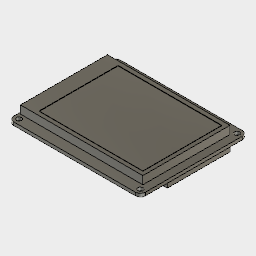
3315 2.4in TFT Feather Wing (Autodesk Fusion 360 design; units mm, degrees)
Autodesk Fusion 360 part; units mm, degrees
note: some values were not read from the file. Set by a fixed rule: which sketch regions a step uses.
sketch "pcb" plane through (0, 0, 0) normal (0, 0, 1) x (1, 0, 0)
  line L0 (0, 0) -> (64.77, 0)
  line L1 (64.77, 0) -> (64.77, 52.578)
  line L2 (64.77, 52.578) -> (0, 52.578)
  line L3 (0, 52.578) -> (0, 0)
  circle A0 centre (2.54, 50.038) radius 1.27
  line L4 (32.385, 52.578) -> (32.385, 0) construction
  line L5 (0, 26.289) -> (64.77, 26.289) construction
  circle A1 centre (62.23, 50.038) radius 1.27
  circle A2 centre (2.54, 2.54) radius 1.27
  circle A3 centre (62.23, 2.54) radius 1.27
  dimension "d1" = 64.77
  dimension "d2" = 52.578
  dimension "d3" = 2.54
  dimension "d4" = 2.54
  dimension "d5" = 2.54
  measures "d1" distance of L1.end L2.end
  measures "d2" distance of L0.start L2.end
  measures "d3" diameter of A0
  measures "d4" distance of L3 A0.centre
  measures "d5" distance of L2 A0.centre
extrude "Extrude1" add sketch "pcb" along normal blind 1.6 makes body 1
fillet "Fillet1" radius 2.54 4 edges at (64.77, 0, 0.8) (0, 0, 0.8) (0, 52.578, 0.8) (64.77, 52.578, 0.8) on bodies 1
sketch "bottom" plane through (0, 0, 0) normal (0, 0, -1) x (1, 0, 0)
  circle A0 centre (62.23, -50.038) radius 1.27
  circle A1 centre (2.54, -2.54) radius 1.27
  circle A2 centre (62.23, -2.54) radius 1.27
  circle A3 centre (2.54, -50.038) radius 1.27
  arc A4 (62.23, -52.578) -> (64.77, -50.038) centre (62.23, -50.038) ccw
  line L0 (64.77, -50.038) -> (64.77, -2.54)
  arc A5 (64.77, -2.54) -> (62.23, 0) centre (62.23, -2.54) ccw
  line L1 (62.23, 0) -> (2.54, 0)
  arc A6 (2.54, 0) -> (0, -2.54) centre (2.54, -2.54) ccw
  line L2 (0, -2.54) -> (0, -50.038)
  arc A7 (0, -50.038) -> (2.54, -52.578) centre (2.54, -50.038) ccw
  line L3 (2.54, -52.578) -> (62.23, -52.578)
  line L4 (62.97, -45.978) -> (57.97, -45.978)
  line L5 (57.97, -45.978) -> (57.97, -14.978)
  line L6 (57.97, -14.978) -> (62.97, -14.978)
  line L7 (62.97, -14.978) -> (62.97, -45.978)
  line L8 (40.17, -45.978) -> (35.17, -45.978)
  line L9 (35.17, -45.978) -> (35.17, -4.978)
  line L10 (35.17, -4.978) -> (40.17, -4.978)
  line L11 (40.17, -4.978) -> (40.17, -45.978)
  line L12 (1.6, -6.8) -> (7.6, -6.8)
  line L13 (7.6, -6.8) -> (7.6, -12.8)
  line L14 (7.6, -12.8) -> (1.6, -12.8)
  line L15 (1.6, -12.8) -> (1.6, -6.8)
  line L16 (1.6, -6.8) -> (7.6, -12.8) construction
  line L17 (7.6, -6.8) -> (1.6, -12.8) construction
  circle A8 centre (4.6, -9.8) radius 1.5
  line L18 (5.5, -17.4) -> (2, -17.4)
  line L19 (2, -17.4) -> (2, -24.4)
  line L20 (2, -24.4) -> (5.5, -24.4)
  line L21 (5.5, -24.4) -> (5.5, -17.4)
  line L22 (15.5, -43.978) -> (0, -43.978)
  line L23 (0, -43.978) -> (0, -29.978)
  line L24 (0, -29.978) -> (15.5, -29.978)
  line L25 (15.5, -29.978) -> (15.5, -43.978)
  point P0 (4.6, -9.8)
  dimension "d9" = 5
  dimension "d10" = 5
  dimension "d11" = 31
  dimension "d12" = 41
  dimension "d13" = 6.6
  dimension "d14" = 6.6
  dimension "d15" = 1.8
  dimension "d16" = 17.8
  dimension "d19" = 6
  dimension "d20" = 6
  dimension "d21" = 6.8
  dimension "d22" = 1.6
  dimension "d23" = 3
  dimension "d28" = 3.5
  dimension "d29" = 7
  dimension "d30" = 2
  dimension "d31" = 17.4
  dimension "d32" = 15.5
  dimension "d33" = 14
  dimension "d34" = 8.6
  measures "d9" distance of L5.end L6.end
  measures "d10" distance of L9.end L10.end
  measures "d11" distance of L4.start L6.end
  measures "d12" distance of L8.start L10.end
  measures "d13" distance of L3 L4
  measures "d14" distance of L3 L8
  measures "d15" distance of L0 L7
  measures "d16" distance of L5 L11
  measures "d19" distance of L13.end L14.end
  measures "d20" distance of L12.end L13.end
  measures "d21" distance of L1 L12
  measures "d22" distance of L2 L15
  measures "d23" diameter of A8
  measures "d28" distance of L18.start L18.end
  measures "d29" distance of L18.start L20.end
  measures "d30" distance of L2 L19
  measures "d31" distance of L1 L18
  measures "d32" distance of L22.start L22.end
  measures "d33" distance of L22.start L24.end
  measures "d34" distance of L3 L22
extrude "Extrude2" add sketch "bottom" along normal blind 3.9 separate body contours L4 L5 L6 L7 | L8 L9 L10 L11 makes body 2 at (61.3033, 25.3113, 0) makes body 3 at (38.5033, 32.3113, 0)
extrude "Extrude3" add sketch "bottom" along normal blind 1.8 separate body contours L12 L13 L14 L15 | A8 makes body 4
extrude "Extrude4" add sketch "bottom" along normal blind 3 contours A8 bodies 4
extrude "Extrude5" add sketch "bottom" along normal blind 1.4 separate body contours L18 L19 L20 L21 makes body 5
extrude "Extrude6" add sketch "bottom" along normal blind 1.7 separate body contours L2 L22 L23 L24 L25 makes body 6
sketch "microSD" plane through (0, 0, -1.7) normal (0, 0, -1) x (1, 0, 0)
  line L0 (15.5, -29.978) -> (0, -29.978)
  line L1 (0, -29.978) -> (0, -43.978)
  line L2 (0, -43.978) -> (15.5, -43.978)
  line L3 (15.5, -43.978) -> (15.5, -29.978)
  circle A0 centre (-8.5, -35.5) radius 11
  dimension "d39" = 22
  measures "d39" diameter of A0
extrude "Extrude7" cut sketch "microSD" against normal blind 1.7 contours L0 L1 A0 picked at (0.2923, -37.9037) bodies 6
sketch "switch" plane through (0, 0, -1.4) normal (0, 0, -1) x (1, 0, 0)
  line L0 (5.5, -24.4) -> (5.5, -17.4)
  line L1 (5.5, -17.4) -> (2, -17.4)
  line L2 (2, -17.4) -> (2, -24.4)
  line L3 (2, -24.4) -> (5.5, -24.4)
  line L4 (2, -20.9) -> (5.5, -20.9)
  line L5 (2, -19.4) -> (3, -19.4)
  line L6 (3, -19.4) -> (3, -22.4)
  line L7 (3, -22.4) -> (2, -22.4)
  line L8 (2, -22.4) -> (2, -19.4)
  line L9 (3, -20.9) -> (2, -20.9) construction
  dimension "d42" = 3
  dimension "d43" = 1
  measures "d42" distance of L5.end L6.end
  measures "d43" distance of L6.end L7.end
extrude "Extrude8" add sketch "switch" along normal blind 1 contours L2 L4 L6 L7 L8 bodies 5
sketch "display" plane through (0, 0, 1.6) normal (0, 0, 1) x (-1, 0, 0)
  arc A0 (-64.77, -50.038) -> (-62.23, -52.578) centre (-62.23, -50.038) ccw
  line L0 (-62.23, -52.578) -> (-2.54, -52.578)
  arc A1 (-2.54, -52.578) -> (0, -50.038) centre (-2.54, -50.038) ccw
  line L1 (0, -50.038) -> (0, -2.54)
  arc A2 (0, -2.54) -> (-2.54, 0) centre (-2.54, -2.54) ccw
  line L2 (-2.54, 0) -> (-62.23, 0)
  arc A3 (-62.23, 0) -> (-64.77, -2.54) centre (-62.23, -2.54) ccw
  line L3 (-64.77, -2.54) -> (-64.77, -50.038)
  circle A4 centre (-62.23, -50.038) radius 1.27
  circle A5 centre (-2.54, -2.54) radius 1.27
  circle A6 centre (-62.23, -2.54) radius 1.27
  circle A7 centre (-2.54, -50.038) radius 1.27
  line L4 (-0.8, -47.778) -> (-61, -47.778)
  line L5 (-61, -47.778) -> (-61, -4.978)
  line L6 (-61, -4.978) -> (-0.8, -4.978)
  line L7 (-0.8, -4.978) -> (-0.8, -47.778)
  dimension "d46" = 60.2
  dimension "d47" = 42.8
  dimension "d48" = 4.8
  dimension "d49" = 0.8
  measures "d46" distance of L4.start L4.end
  measures "d47" distance of L4.start L6.end
  measures "d48" distance of L0 L4
  measures "d49" distance of L1 L7
extrude "Extrude9" add sketch "display" along normal blind 3.9 separate body contours L4 L5 L6 L7 makes body 7
sketch "view" plane through (0, 0, 5.5) normal (0, 0, 1) x (-1, 0, 0)
  line L0 (-0.8, -4.978) -> (-61, -4.978)
  line L1 (-61, -4.978) -> (-61, -47.778)
  line L2 (-61, -47.778) -> (-0.8, -47.778)
  line L3 (-0.8, -47.778) -> (-0.8, -4.978)
  line L4 (-8, -45.778) -> (-59, -45.778)
  line L5 (-59, -45.778) -> (-59, -6.978)
  line L6 (-59, -6.978) -> (-8, -6.978)
  line L7 (-8, -6.978) -> (-8, -45.778)
  dimension "d52" = 2
  dimension "d53" = 2
  dimension "d54" = 2
  dimension "d55" = 7.2
  measures "d52" distance of L0 L6
  measures "d53" distance of L1 L5
  measures "d54" distance of L2 L4
  measures "d55" distance of L3 L7
extrude "Extrude10" cut sketch "view" against normal blind 0.2 contours L4 L5 L6 L7 bodies 7
ref_plane "WorkPlane1" through (30.9, 26.378, 5.7) normal (0, 0, 1) x (1, 0, 0) in component "mount"
sketch "Sketch1" plane through (30.9, 26.378, 5.7) normal (0, 0, 1) x (1, 0, 0) in component "mount"
  line L0 (-32.9, 28.2) -> (35.87, 28.2)
  line L1 (35.87, 28.2) -> (35.87, -28.378)
  line L2 (35.87, -28.378) -> (-32.9, -28.378)
  line L3 (-32.9, -28.378) -> (-32.9, 28.2)
  line L4 (31.33, 26.2) -> (-28.36, 26.2) construction
  line L5 (33.87, -23.838) -> (33.87, 23.66) construction
  line L6 (-30.9, 23.66) -> (-30.9, -23.838) construction
  line L7 (-28.36, -26.378) -> (31.33, -26.378) construction
  line L8 (-22.9, -19.4) -> (28.1, -19.4)
  line L9 (28.1, -19.4) -> (28.1, 19.4)
  line L10 (28.1, 19.4) -> (-22.9, 19.4)
  line L11 (-22.9, 19.4) -> (-22.9, -19.4)
  circle A0 centre (-28.36, -23.838) radius 1.27
  circle A1 centre (31.33, -23.838) radius 1.27
  circle A2 centre (31.33, 23.66) radius 1.27
  circle A3 centre (-28.36, 23.66) radius 1.27
  line L12 (30.1, -21.4) -> (-30.1, -21.4) construction
  line L13 (-30.1, -21.4) -> (-30.1, 21.4) construction
  line L14 (-30.1, 21.4) -> (30.1, 21.4) construction
  line L15 (30.1, 21.4) -> (30.1, -21.4) construction
  circle A4 centre (-28.36, -23.838) radius 2.77
  circle A5 centre (31.33, 23.66) radius 2.77
  circle A6 centre (-28.36, 23.66) radius 2.77
  line L16 (-30.7, -22) -> (-30.7, 22)
  line L17 (-30.7, 22) -> (30.7, 22)
  line L18 (30.7, 22) -> (30.7, -22)
  line L19 (30.7, -22) -> (-30.7, -22)
  circle A7 centre (31.33, -23.838) radius 2.77
  point P0 (30.06, -23.838)
  dimension "d59" = 2
  dimension "d60" = 2
  dimension "d61" = 2
  dimension "d62" = 2
  dimension "d65" = 1.5
  dimension "d66" = 1.5
  dimension "d67" = 1.5
  dimension "d68" = 1.5
  dimension "d74" = 0.6
  measures "d59" distance of L0 L4
  measures "d60" distance of L1 L5
  measures "d61" distance of L3 L6
  measures "d62" distance of L2 L7
extrude "Extrude1'" add sketch "Sketch1" along normal blind 1 separate body contours L0 L1 L2 L3 | A0 | A1 | A2 | A3 | A4 L19 | A4 L19 | A4 A5 A6 L16 L17 L18 L19 A7 | L18 L19 A7 | L18 L19 A7 | A5 L17 L18 | A5 L17 L18 | A6 L17 | A6 L17 makes body 8 in component "mount"
extrude "Extrude2'" add sketch "Sketch1" against normal up to surface (4.1 mm away) contours A0 | A1 | A2 | A3 | A4 L19 | A4 L19 | L18 L19 A7 | L18 L19 A7 | A5 L17 L18 | A5 L17 L18 | A6 L17 | A6 L17 bodies 8 in component "mount"
extrude "Extrude3'" add sketch "Sketch1" against normal blind 6.5 contours A0 | A1 | A2 | A3 bodies 8 in component "mount"
fillet "Fillet1'" radius 2.54 4 edges at (-2, -2, 6.2) (66.77, -2, 6.2) (-2, 54.578, 6.2) (66.77, 54.578, 6.2) on bodies 8 in component "mount"
extrude "Extrude4'" cut sketch "Sketch1" against normal blind 5 contours A4 L19 | A4 A5 A6 L16 L17 L18 L19 A7 | L18 L19 A7 | A5 L17 L18 | A6 L17 picked at (-28.2304, -21.6985) picked at (30.5911, -21.4597) picked at (30.5768, 21.3464) picked at (-27.9175, 21.7429) bodies 8 in component "mount"
component "mount" placed x (1, 0, 0) y (0, 1, 0) z (0, 0, 1) at (0, 0, 0)
named bodies: "pcb", "header medium", "header long", "pushbutton", "microSD", "switch", "display"
